Autodesk Inventor part; units mm, degrees
(part 2 of 2)
  line L111 (-7.2782, 22.2196) -> (-7.2782, 21.0994)
  arc A139 (-6.6783, 17.8482) -> (-5.3536, 18.9958) centre (-6.7426, 19.2608) ccw
  arc A140 (-5.4999, 21.453) -> (-6.4187, 22.2196) centre (-6.6691, 20.9857) ccw
  arc A141 (-5.3536, 18.9958) -> (-5.4999, 21.453) centre (-9.1247, 20.0042) ccw
  line L112 (-6.4187, 22.2196) -> (-7.2782, 22.2196)
  circle A142 centre (-10.9934, 23.3802) radius 0.3922
  circle A143 centre (-8.5106, 16.5617) radius 0.4142
  spline S0 degree 2 poles (-54.0773, 84.6678) (-54.4478, 84.6678) (-55.1805, 84.4867) (-55.5346, 84.3467) knots 0 0 0 1 2 2 2
  spline S1 degree 2 poles (-55.5346, 84.3467) (-55.8639, 84.2067) (-56.3497, 83.9103) (-56.5391, 83.7786) knots 0 0 0 1 2 2 2
  line L113 (-56.5391, 83.7786) -> (-56.6214, 83.7786)
  line L114 (-56.6214, 83.7786) -> (-56.6214, 85.2194)
  spline S2 degree 2 poles (-56.6214, 85.2194) (-56.1768, 85.4582) (-54.6536, 85.8452) (-53.9702, 85.8452) knots 0 0 0 1 2 2 2
  spline S3 degree 2 poles (-53.9702, 85.8452) (-53.2786, 85.8452) (-52.2495, 85.5652) (-51.8296, 85.2688) knots 0 0 0 1 2 2 2
  spline S4 degree 2 poles (-51.8296, 85.2688) (-51.385, 84.9477) (-50.9239, 84.0174) (-50.9239, 83.3916) knots 0 0 0 1 2 2 2
  spline S5 degree 2 poles (-50.9239, 83.3916) (-50.9239, 82.5518) (-52.0272, 81.2839) (-52.8011, 81.1192) knots 0 0 0 1 2 2 2
  line L115 (-52.8011, 81.1192) -> (-52.8011, 81.0204)
  spline S6 degree 2 poles (-52.8011, 81.0204) (-52.48, 80.9545) (-51.7472, 80.6581) (-51.4344, 80.3617) knots 0 0 0 1 2 2 2
  spline S7 degree 2 poles (-51.4344, 80.3617) (-51.1215, 80.0736) (-50.7263, 79.1514) (-50.7263, 78.4845) knots 0 0 0 1 2 2 2
  spline S8 degree 2 poles (-50.7263, 78.4845) (-50.7263, 77.8012) (-51.1956, 76.6403) (-51.6237, 76.1956) knots 0 0 0 1 2 2 2
  spline S9 degree 2 poles (-51.6237, 76.1956) (-52.0683, 75.7346) (-53.328, 75.257) (-54.1267, 75.257) knots 0 0 0 1 2 2 2
  spline S10 degree 2 poles (-54.1267, 75.257) (-54.8924, 75.257) (-56.3909, 75.6275) (-56.9013, 75.8828) knots 0 0 0 1 2 2 2
  line L116 (-56.9013, 75.8828) -> (-56.9013, 77.3236)
  line L117 (-56.9013, 77.3236) -> (-56.8025, 77.3236)
  spline S11 degree 2 poles (-56.8025, 77.3236) (-56.3744, 77.0108) (-54.9253, 76.4344) (-54.209, 76.4344) knots 0 0 0 1 2 2 2
  spline S12 degree 2 poles (-54.209, 76.4344) (-53.7891, 76.4344) (-52.9493, 76.6979) (-52.6694, 77.0025) knots 0 0 0 1 2 2 2
  spline S13 degree 2 poles (-52.6694, 77.0025) (-52.3977, 77.3072) (-52.1095, 78.0317) (-52.1095, 78.5833) knots 0 0 0 1 2 2 2
  spline S14 degree 2 poles (-52.1095, 78.5833) (-52.1095, 79.135) (-52.4306, 79.8513) (-52.7188, 80.0571) knots 0 0 0 1 2 2 2
  spline S15 degree 2 poles (-52.7188, 80.0571) (-53.0069, 80.2629) (-53.7891, 80.4194) (-54.2502, 80.4194) knots 0 0 0 1 2 2 2
  line L118 (-54.2502, 80.4194) -> (-54.8265, 80.4194)
  line L119 (-54.8265, 80.4194) -> (-54.8265, 81.5474)
  line L120 (-54.8265, 81.5474) -> (-54.3737, 81.5474)
  spline S16 degree 2 poles (-54.3737, 81.5474) (-53.4598, 81.5474) (-52.3071, 82.4201) (-52.3071, 83.2517) knots 0 0 0 1 2 2 2
  spline S17 degree 2 poles (-52.3071, 83.2517) (-52.3071, 83.6386) (-52.6035, 84.1903) (-52.8423, 84.3549) knots 0 0 0 1 2 2 2
  spline S18 degree 2 poles (-52.8423, 84.3549) (-53.0975, 84.5278) (-53.7232, 84.6678) (-54.0773, 84.6678) knots 0 0 0 1 2 2 2
  spline S19 degree 2 poles (-9.4227, 4.5768) (-9.0522, 4.5768) (-8.3195, 4.7579) (-7.9654, 4.8979) knots 0 0 0 1 2 2 2
  spline S20 degree 2 poles (-7.9654, 4.8979) (-7.6361, 5.0378) (-7.1503, 5.3342) (-6.9609, 5.466) knots 0 0 0 1 2 2 2
  line L121 (-6.9609, 5.466) -> (-6.8786, 5.466)
  line L122 (-6.8786, 5.466) -> (-6.8786, 4.0251)
  spline S21 degree 2 poles (-6.8786, 4.0251) (-7.3232, 3.7864) (-8.8464, 3.3994) (-9.5298, 3.3994) knots 0 0 0 1 2 2 2
  spline S22 degree 2 poles (-9.5298, 3.3994) (-10.2214, 3.3994) (-11.2505, 3.6793) (-11.6704, 3.9757) knots 0 0 0 1 2 2 2
  spline S23 degree 2 poles (-11.6704, 3.9757) (-12.115, 4.2968) (-12.5761, 5.2272) (-12.5761, 5.8529) knots 0 0 0 1 2 2 2
  spline S24 degree 2 poles (-12.5761, 5.8529) (-12.5761, 6.6927) (-11.4728, 7.9607) (-10.6989, 8.1254) knots 0 0 0 1 2 2 2
  line L123 (-10.6989, 8.1254) -> (-10.6989, 8.2242)
  spline S25 degree 2 poles (-10.6989, 8.2242) (-11.02, 8.29) (-11.7528, 8.5864) (-12.0656, 8.8828) knots 0 0 0 1 2 2 2
  spline S26 degree 2 poles (-12.0656, 8.8828) (-12.3785, 9.171) (-12.7737, 10.0931) (-12.7737, 10.76) knots 0 0 0 1 2 2 2
  spline S27 degree 2 poles (-12.7737, 10.76) (-12.7737, 11.4434) (-12.3044, 12.6043) (-11.8763, 13.0489) knots 0 0 0 1 2 2 2
  spline S28 degree 2 poles (-11.8763, 13.0489) (-11.4317, 13.51) (-10.172, 13.9875) (-9.3733, 13.9875) knots 0 0 0 1 2 2 2
  spline S29 degree 2 poles (-9.3733, 13.9875) (-8.6076, 13.9875) (-7.1091, 13.617) (-6.5987, 13.3618) knots 0 0 0 1 2 2 2
  line L124 (-6.5987, 13.3618) -> (-6.5987, 11.921)
  line L125 (-6.5987, 11.921) -> (-6.6975, 11.921)
  spline S30 degree 2 poles (-6.6975, 11.921) (-7.1256, 12.2338) (-8.5747, 12.8102) (-9.291, 12.8102) knots 0 0 0 1 2 2 2
  spline S31 degree 2 poles (-9.291, 12.8102) (-9.7109, 12.8102) (-10.5507, 12.5467) (-10.8306, 12.2421) knots 0 0 0 1 2 2 2
  spline S32 degree 2 poles (-10.8306, 12.2421) (-11.1023, 11.9374) (-11.3905, 11.2129) (-11.3905, 10.6612) knots 0 0 0 1 2 2 2
  spline S33 degree 2 poles (-11.3905, 10.6612) (-11.3905, 10.1096) (-11.0694, 9.3933) (-10.7812, 9.1875) knots 0 0 0 1 2 2 2
  spline S34 degree 2 poles (-10.7812, 9.1875) (-10.4931, 8.9816) (-9.7109, 8.8252) (-9.2498, 8.8252) knots 0 0 0 1 2 2 2
  line L126 (-9.2498, 8.8252) -> (-8.6735, 8.8252)
  line L127 (-8.6735, 8.8252) -> (-8.6735, 7.6972)
  line L128 (-8.6735, 7.6972) -> (-9.1263, 7.6972)
  spline S35 degree 2 poles (-9.1263, 7.6972) (-10.0402, 7.6972) (-11.1929, 6.8245) (-11.1929, 5.9929) knots 0 0 0 1 2 2 2
  spline S36 degree 2 poles (-11.1929, 5.9929) (-11.1929, 5.6059) (-10.8965, 5.0543) (-10.6577, 4.8896) knots 0 0 0 1 2 2 2
  spline S37 degree 2 poles (-10.6577, 4.8896) (-10.4025, 4.7167) (-9.7768, 4.5768) (-9.4227, 4.5768) knots 0 0 0 1 2 2 2
  spline S38 degree 2 poles (-54.0773, 84.6678) (-54.4478, 84.6678) (-55.1805, 84.4867) (-55.5346, 84.3467) knots 0 0 0 1 2 2 2
  spline S39 degree 2 poles (-55.5346, 84.3467) (-55.8639, 84.2067) (-56.3497, 83.9103) (-56.5391, 83.7786) knots 0 0 0 1 2 2 2
  line L129 (-56.5391, 83.7786) -> (-56.6214, 83.7786)
  line L130 (-56.6214, 83.7786) -> (-56.6214, 85.2194)
  spline S40 degree 2 poles (-56.6214, 85.2194) (-56.1768, 85.4582) (-54.6536, 85.8452) (-53.9702, 85.8452) knots 0 0 0 1 2 2 2
  spline S41 degree 2 poles (-53.9702, 85.8452) (-53.2786, 85.8452) (-52.2495, 85.5652) (-51.8296, 85.2688) knots 0 0 0 1 2 2 2
  spline S42 degree 2 poles (-51.8296, 85.2688) (-51.385, 84.9477) (-50.9239, 84.0174) (-50.9239, 83.3916) knots 0 0 0 1 2 2 2
  spline S43 degree 2 poles (-50.9239, 83.3916) (-50.9239, 82.5518) (-52.0272, 81.2839) (-52.8011, 81.1192) knots 0 0 0 1 2 2 2
  line L131 (-52.8011, 81.1192) -> (-52.8011, 81.0204)
  spline S44 degree 2 poles (-52.8011, 81.0204) (-52.48, 80.9545) (-51.7472, 80.6581) (-51.4344, 80.3617) knots 0 0 0 1 2 2 2
  spline S45 degree 2 poles (-51.4344, 80.3617) (-51.1215, 80.0736) (-50.7263, 79.1514) (-50.7263, 78.4845) knots 0 0 0 1 2 2 2
  spline S46 degree 2 poles (-50.7263, 78.4845) (-50.7263, 77.8012) (-51.1956, 76.6403) (-51.6237, 76.1956) knots 0 0 0 1 2 2 2
  spline S47 degree 2 poles (-51.6237, 76.1956) (-52.0683, 75.7346) (-53.328, 75.257) (-54.1267, 75.257) knots 0 0 0 1 2 2 2
  spline S48 degree 2 poles (-54.1267, 75.257) (-54.8924, 75.257) (-56.3909, 75.6275) (-56.9013, 75.8828) knots 0 0 0 1 2 2 2
  line L132 (-56.9013, 75.8828) -> (-56.9013, 77.3236)
  line L133 (-56.9013, 77.3236) -> (-56.8025, 77.3236)
  spline S49 degree 2 poles (-56.8025, 77.3236) (-56.3744, 77.0108) (-54.9253, 76.4344) (-54.209, 76.4344) knots 0 0 0 1 2 2 2
  spline S50 degree 2 poles (-54.209, 76.4344) (-53.7891, 76.4344) (-52.9493, 76.6979) (-52.6694, 77.0025) knots 0 0 0 1 2 2 2
  spline S51 degree 2 poles (-52.6694, 77.0025) (-52.3977, 77.3072) (-52.1095, 78.0317) (-52.1095, 78.5833) knots 0 0 0 1 2 2 2
  spline S52 degree 2 poles (-52.1095, 78.5833) (-52.1095, 79.135) (-52.4306, 79.8513) (-52.7188, 80.0571) knots 0 0 0 1 2 2 2
  spline S53 degree 2 poles (-52.7188, 80.0571) (-53.0069, 80.2629) (-53.7891, 80.4194) (-54.2502, 80.4194) knots 0 0 0 1 2 2 2
  line L134 (-54.2502, 80.4194) -> (-54.8265, 80.4194)
  line L135 (-54.8265, 80.4194) -> (-54.8265, 81.5474)
  line L136 (-54.8265, 81.5474) -> (-54.3737, 81.5474)
  spline S54 degree 2 poles (-54.3737, 81.5474) (-53.4598, 81.5474) (-52.3071, 82.4201) (-52.3071, 83.2517) knots 0 0 0 1 2 2 2
  spline S55 degree 2 poles (-52.3071, 83.2517) (-52.3071, 83.6386) (-52.6035, 84.1903) (-52.8423, 84.3549) knots 0 0 0 1 2 2 2
  spline S56 degree 2 poles (-52.8423, 84.3549) (-53.0975, 84.5278) (-53.7232, 84.6678) (-54.0773, 84.6678) knots 0 0 0 1 2 2 2
  spline S57 degree 2 poles (-9.4227, 4.5768) (-9.0522, 4.5768) (-8.3195, 4.7579) (-7.9654, 4.8979) knots 0 0 0 1 2 2 2
  spline S58 degree 2 poles (-7.9654, 4.8979) (-7.6361, 5.0378) (-7.1503, 5.3342) (-6.9609, 5.466) knots 0 0 0 1 2 2 2
  line L137 (-6.9609, 5.466) -> (-6.8786, 5.466)
  line L138 (-6.8786, 5.466) -> (-6.8786, 4.0251)
  spline S59 degree 2 poles (-6.8786, 4.0251) (-7.3232, 3.7864) (-8.8464, 3.3994) (-9.5298, 3.3994) knots 0 0 0 1 2 2 2
  spline S60 degree 2 poles (-9.5298, 3.3994) (-10.2214, 3.3994) (-11.2505, 3.6793) (-11.6704, 3.9757) knots 0 0 0 1 2 2 2
  spline S61 degree 2 poles (-11.6704, 3.9757) (-12.115, 4.2968) (-12.5761, 5.2272) (-12.5761, 5.8529) knots 0 0 0 1 2 2 2
  spline S62 degree 2 poles (-12.5761, 5.8529) (-12.5761, 6.6927) (-11.4728, 7.9607) (-10.6989, 8.1254) knots 0 0 0 1 2 2 2
  line L139 (-10.6989, 8.1254) -> (-10.6989, 8.2242)
  spline S63 degree 2 poles (-10.6989, 8.2242) (-11.02, 8.29) (-11.7528, 8.5864) (-12.0656, 8.8828) knots 0 0 0 1 2 2 2
  spline S64 degree 2 poles (-12.0656, 8.8828) (-12.3785, 9.171) (-12.7737, 10.0931) (-12.7737, 10.76) knots 0 0 0 1 2 2 2
  spline S65 degree 2 poles (-12.7737, 10.76) (-12.7737, 11.4434) (-12.3044, 12.6043) (-11.8763, 13.0489) knots 0 0 0 1 2 2 2
  spline S66 degree 2 poles (-11.8763, 13.0489) (-11.4317, 13.51) (-10.172, 13.9875) (-9.3733, 13.9875) knots 0 0 0 1 2 2 2
  spline S67 degree 2 poles (-9.3733, 13.9875) (-8.6076, 13.9875) (-7.1091, 13.617) (-6.5987, 13.3618) knots 0 0 0 1 2 2 2
  line L140 (-6.5987, 13.3618) -> (-6.5987, 11.921)
  line L141 (-6.5987, 11.921) -> (-6.6975, 11.921)
  spline S68 degree 2 poles (-6.6975, 11.921) (-7.1256, 12.2338) (-8.5747, 12.8102) (-9.291, 12.8102) knots 0 0 0 1 2 2 2
  spline S69 degree 2 poles (-9.291, 12.8102) (-9.7109, 12.8102) (-10.5507, 12.5467) (-10.8306, 12.2421) knots 0 0 0 1 2 2 2
  spline S70 degree 2 poles (-10.8306, 12.2421) (-11.1023, 11.9374) (-11.3905, 11.2129) (-11.3905, 10.6612) knots 0 0 0 1 2 2 2
  spline S71 degree 2 poles (-11.3905, 10.6612) (-11.3905, 10.1096) (-11.0694, 9.3933) (-10.7812, 9.1875) knots 0 0 0 1 2 2 2
  spline S72 degree 2 poles (-10.7812, 9.1875) (-10.4931, 8.9816) (-9.7109, 8.8252) (-9.2498, 8.8252) knots 0 0 0 1 2 2 2
  line L142 (-9.2498, 8.8252) -> (-8.6735, 8.8252)
  line L143 (-8.6735, 8.8252) -> (-8.6735, 7.6972)
  line L144 (-8.6735, 7.6972) -> (-9.1263, 7.6972)
  spline S73 degree 2 poles (-9.1263, 7.6972) (-10.0402, 7.6972) (-11.1929, 6.8245) (-11.1929, 5.9929) knots 0 0 0 1 2 2 2
  spline S74 degree 2 poles (-11.1929, 5.9929) (-11.1929, 5.6059) (-10.8965, 5.0543) (-10.6577, 4.8896) knots 0 0 0 1 2 2 2
  spline S75 degree 2 poles (-10.6577, 4.8896) (-10.4025, 4.7167) (-9.7768, 4.5768) (-9.4227, 4.5768) knots 0 0 0 1 2 2 2
  point P0 (-31.75, 68.8958)
  point P1 (-31.75, 44.45)
  point P2 (-31.75, 20.0009)
  point P3 (-53.7479, 68.8958)
  point P4 (-9.7521, 20.0042)
  point P5 (-13.4723, 102.9238)
  point P6 (-31.75, 68.8958)
  point P7 (-31.75, 44.45)
  point P8 (-31.75, 20.0009)
  point P9 (-53.7479, 68.8958)
  point P10 (-9.7521, 20.0042)
  dimension "d103" = 8.4153
  dimension "d105" = 0.508
  dimension "d106" = 0.508
  constraints: 264 point on circle, 202 end point, 144 centre point, 24 perpendicular, 24 tangent, 10 vertical, 5 horizontal, 2 midpoint, 1 parallel, 4 other
  measures "d103" distance of L12.end L14.start
  measures "d105" distance between parallel lines of L15 L7
  measures "d106" distance between parallel lines of L16 L11
extrude "Extrusion20" add sketch "Sketch17" along normal blind 0.4 contours L40 A34 A33 A32 L39 L38 L37 L36 A31 A30 A29 A28 A27 L35 A26 L34 A25 A24 L33 | L56 A58 A57 A56 L55 L54 L53 L52 A55 A54 A53 A52 A51 L51 A50 L50 A49 A48 L49 | L72 A82 A81 A80 L71 L70 L69 L68 A79 A78 A77 A76 A75 L67 A74 L66 A73 A72 L65 | L88 A106 A105 A104 L87 L86 L85 L84 A103 A102 A101 A100 A99 L83 A98 L82 A97 A96 L81 | L108 A137 A136 L111 L112 A140 A141 A139 L109 L105 L107 L110 A135 A134 A132 A138 A133 L106 A131 | S0 S1 L113 L114 S2 S3 S4 S5 L115 S6 S7 S8 S9 S10 L116 L117 S11 S12 S13 S14 S15 L118 L119 L120 S16 S17 S18 | S19 S20 L121 L122 S21 S22 S23 S24 L123 S25 S26 S27 S28 S29 L124 L125 S30 S31 S32 S33 S34 L126 L127 L128 S35 S36 S37 bodies 1
sketch "Sketch18" plane through (0, 0, -0.2) normal (0, 0, -1) x (-1, 0, 0)
  line L0 (0, 0) -> (-63.5, 0)
  line L1 (-63.5, 0) -> (-63.5, 88.9)
  line L2 (-63.5, 88.9) -> (0, 88.9)
  line L3 (0, 88.9) -> (0, 0)
  constraints: 8 end point, 2 parallel, 1 horizontal, 1 perpendicular
extrude "Extrusion21" add sketch "Sketch18" along normal blind 0.4 bodies 3
fillet "Fillet2" radius 3.175 8 edges at (63.5, 0, 0.2) (63.5, 88.9, 0.2) (0, 0, 0.2) (0, 88.9, 0.2) (63.5, 0, -0.3) (63.5, 88.9, -0.3) (0, 0, -0.3) (0, 88.9, -0.3)
extrude "Extrusion22" cut sketch "Sketch17" along normal blind 0.4 contours L40 A34 A33 A32 L39 L38 L37 L36 A31 A30 A29 A28 A27 L35 A26 L34 A25 A24 L33 | L44 A41 A40 L47 L48 A44 A45 A43 L45 L41 L43 L46 A39 A38 A36 A42 A37 L42 A35 | L56 A58 A57 A56 L55 L54 L53 L52 A55 A54 A53 A52 A51 L51 A50 L50 A49 A48 L49 | L60 A65 A64 L63 L64 A68 A69 A67 L61 L57 L59 L62 A63 A62 A60 A66 A61 L58 A59 | L72 A82 A81 A80 L71 L70 L69 L68 A79 A78 A77 A76 A75 L67 A74 L66 A73 A72 L65 | L76 A89 A88 L79 L80 A92 A93 A91 L77 L73 L75 L78 A87 A86 A84 A90 A85 L74 A83 | L88 A106 A105 A104 L87 L86 L85 L84 A103 A102 A101 A100 A99 L83 A98 L82 A97 A96 L81 | L92 A113 A112 L95 L96 A116 A117 A115 L93 L89 L91 L94 A111 A110 A108 A114 A109 L90 A107 | L104 A130 A129 A128 L103 L102 L101 L100 A127 A126 A125 A124 A123 L99 A122 L98 A121 A120 L97 | L108 A137 A136 L111 L112 A140 A141 A139 L109 L105 L107 L110 A135 A134 A132 A138 A133 L106 A131 | S0 S1 L113 L114 S2 S3 S4 S5 L115 S6 S7 S8 S9 S10 L116 L117 S11 S12 S13 S14 S15 L118 L119 L120 S16 S17 S18 | S19 S20 L121 L122 S21 S22 S23 S24 L123 S25 S26 S27 S28 S29 L124 L125 S30 S31 S32 S33 S34 L126 L127 L128 S35 S36 S37 bodies 3
extrude "Extrusion23" add sketch "Sketch17" along normal blind 0.4 contours L44 A41 A40 L47 L48 A44 A45 A43 L45 L41 L43 L46 A39 A38 A36 A42 A37 L42 A35 | L60 A65 A64 L63 L64 A68 A69 A67 L61 L57 L59 L62 A63 A62 A60 A66 A61 L58 A59 | L76 A89 A88 L79 L80 A92 A93 A91 L77 L73 L75 L78 A87 A86 A84 A90 A85 L74 A83 | L92 A113 A112 L95 L96 A116 A117 A115 L93 L89 L91 L94 A111 A110 A108 A114 A109 L90 A107 | L104 A130 A129 A128 L103 L102 L101 L100 A127 A126 A125 A124 A123 L99 A122 L98 A121 A120 L97 bodies 4
